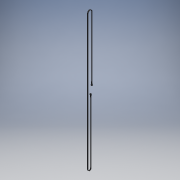
# Autodesk Inventor part: first stage belt
Saved by Autodesk Inventor 2017 SP1 (Build 210196100, 196)
## iProperties
Created: 2018-01-21
Part Number: first stage belt
Material: Rubber
Document SubType Name: Modeling
Designer: Ben
Density: 0.93 g/cm^3
Appearance: Rubber - Black
Mass: 35.5868 g
Surface Area: 562.733 cm^2
Volume: 38.2653 cm^3
Author: Ben
Autodesk Inventor part; units mm, degrees
ref_plane "YZ Plane" through (0, 0, 0) normal (1, 0, 0) x (0, 1, 0)
ref_plane "XZ Plane" through (0, 0, 0) normal (0, 1, 0) x (-1, 0, 0)
ref_plane "XY Plane" through (0, 0, 0) normal (0, 0, 1) x (1, 0, 0)
sketch "Sketch1" plane through (0, 0, 0) normal (1, 0, 0) x (0, 1, 0)
  line L0 (603.25, 0) -> (-603.25, 0)
  line L1 (0, 0) -> (0, -30.1625) construction
  arc A0 (603.25, -34.925) -> (603.25, 0) centre (603.25, -17.4625) ccw
  line L2 (603.25, -34.925) -> (46.592, -34.925)
  arc A1 (-603.25, 0) -> (-603.25, -25.4) centre (-603.25, -12.7) ccw
  line L3 (-603.25, -25.4) -> (-46.592, -25.4)
  arc A2 (32.4346, -31.8247) -> (32.464, -38.0187) centre (31.75, -34.925) ccw
  arc A3 (-32.464, -28.4937) -> (-32.4346, -22.2997) centre (-31.75, -25.4) ccw
  line L4 (46.592, -36.5125) -> (603.25, -36.5125)
  arc A4 (603.25, -36.5125) -> (603.25, 1.5875) centre (603.25, -17.4625) ccw
  line L5 (603.25, 1.5875) -> (-603.25, 1.5875)
  arc A5 (-603.25, 1.5875) -> (-603.25, -26.9875) centre (-603.25, -12.7) ccw
  line L6 (-603.25, -26.9875) -> (-46.592, -26.9875)
  line L7 (31.75, -34.925) -> (-31.75, -25.4) construction
  arc A6 (32.7769, -30.2745) -> (32.821, -39.5655) centre (31.75, -34.925) ccw
  arc A7 (46.592, -34.925) -> (45.164, -35.0876) centre (46.592, -41.275) ccw
  line L8 (45.164, -35.0876) -> (32.464, -38.0187)
  arc A8 (46.592, -36.5125) -> (45.521, -36.6345) centre (46.592, -41.275) ccw
  line L9 (45.521, -36.6345) -> (32.821, -39.5655)
  arc A9 (45.2227, -34.6486) -> (46.592, -34.798) centre (46.592, -28.448) ccw
  line L10 (46.592, -34.798) -> (59.292, -34.798)
  line L11 (45.2227, -34.6486) -> (32.4346, -31.8247)
  line L12 (46.592, -34.798) -> (46.592, -34.925) construction
  line L13 (59.292, -34.798) -> (59.292, -33.2105)
  line L14 (59.292, -33.2105) -> (46.592, -33.2105)
  arc A10 (45.565, -33.0985) -> (46.592, -33.2105) centre (46.592, -28.448) ccw
  line L15 (45.565, -33.0985) -> (32.7769, -30.2745)
  arc A11 (-45.521, -27.1095) -> (-46.592, -26.9875) centre (-46.592, -31.75) ccw
  arc A12 (-45.164, -25.5626) -> (-46.592, -25.4) centre (-46.592, -31.75) ccw
  line L16 (-45.164, -25.5626) -> (-32.464, -28.4937)
  arc A13 (-32.821, -30.0405) -> (-32.7769, -20.7495) centre (-31.75, -25.4) ccw
  line L17 (-32.821, -30.0405) -> (-45.521, -27.1095)
  line L18 (-32.4346, -22.2997) -> (-45.2227, -25.1236)
  arc A14 (-46.592, -25.273) -> (-45.2227, -25.1236) centre (-46.592, -18.923) ccw
  line L19 (-46.592, -25.4) -> (-46.592, -25.273) construction
  line L20 (-46.592, -25.273) -> (-59.292, -25.273)
  line L21 (-59.292, -25.273) -> (-59.292, -23.6855)
  line L22 (-59.292, -23.6855) -> (-46.592, -23.6855)
  arc A15 (-46.592, -23.6855) -> (-45.565, -23.5735) centre (-46.592, -18.923) ccw
  line L23 (-45.565, -23.5735) -> (-32.7769, -20.7495)
  dimension "d1" = 17.4625
  dimension "d2" = 12.7
  dimension "d4" = 6.35
  dimension "d5" = 1.5875
  dimension "d6" = 63.5
  dimension "d7" = 6.35
  dimension "d8" = 12.7
  dimension "d9" = 12.7
  dimension "d10" = 0.127
  dimension "d11" = 6.35
  dimension "d12" = 12.7
  dimension "d13" = 0.127
  dimension "d14" = 12.7
  dimension "d15" = 1206.5
  constraints: 49 end point, 32 point on circle, 26 tangent, 16 centre point, 7 coincident, 6 parallel, 5 horizontal, 5 vertical, 3 equal radius, 2 midpoint, 2 point on line, 1 line through centre, 1 perpendicular, 4 other
  measures "d1" radius of A0
  measures "d2" radius of A1
  measures "d4" diameter of A2
  measures "d5" distance between parallel lines of L5 L0
  measures "d6" horizontal distance of L7.start L7.end
  measures "d7" radius of A7
  measures "d8" horizontal distance of L8.start L8.end
  measures "d9" distance of L10.start L10.end
  measures "d10" distance between parallel lines of L10 L2
  measures "d11" radius of A12
  measures "d12" horizontal distance of L16.start L16.end
  measures "d13" distance of L3.end L19.end
  measures "d14" distance of L19.end L20.end
  measures "d15" horizontal distance of A1.centre A0.centre
extrude "Extrusion1" add sketch "Sketch1" along normal mid plane 9.525
body "Solid1"
